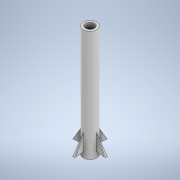
# Autodesk Inventor part: body
Saved by Autodesk Inventor 2022 (Build 260153000, 153)
## iProperties
Created: 2023-01-18
Part Number: body
Material: Generic
Document SubType Name: Modeling
Designer: CLCK
Density: 1 g/cm^3
Appearance: Default
Author: CLCK
Autodesk Inventor part; units mm, degrees
ref_plane "YZ Plane" through (0, 0, 0) normal (1, 0, 0) x (0, 1, 0)
ref_plane "XZ Plane" through (0, 0, 0) normal (0, 1, 0) x (-1, 0, 0)
ref_plane "XY Plane" through (0, 0, 0) normal (0, 0, 1) x (1, 0, 0)
sketch "Sketch2" plane through (0, 0, 0) normal (1, 0, 0) x (0, 1, 0)
  line L0 (50, 4) -> (-50, 4)
  line L1 (-50, 4) -> (-50, -4)
  line L2 (-50, -4) -> (50, -4)
  line L3 (50, -4) -> (50, 4)
  line L4 (50, 4) -> (-50, -4) construction
  line L5 (-50, 4) -> (50, -4) construction
  line L6 (50, 6) -> (-50, 6)
  line L7 (-50, 6) -> (-50, -6)
  line L8 (-50, -6) -> (50, -6)
  line L9 (50, -6) -> (50, 6)
  line L10 (50, 6) -> (-50, -6) construction
  line L11 (-50, 6) -> (50, -6) construction
  line L12 (50, 0) -> (-50, 0)
  point P0 (0, 0)
  dimension "d0" = 100
  dimension "d1" = 8
  dimension "d2" = 100
  dimension "d3" = 12
  constraints: 26 end point, 6 midpoint, 4 parallel, 2 horizontal, 2 perpendicular
  measures "d0" distance of L2.end L1.end
  measures "d1" distance of L1.end L0.end
  measures "d2" distance of L8.end L7.end
  measures "d3" distance of L7.end L6.end
revolve "Revolution1" add sketch "Sketch2" angle 360 about axis through (0, 50, 0) along (0, -1, 0) contours L9 L8 L7 L2
sketch "Sketch4" plane through (0, 0, 0) normal (0, 0, 1) x (1, 0, 0)
  line L0 (6, 50) -> (6, -50) projected
  line L1 (6, -45) -> (6, -30)
  line L2 (6, -30) -> (14.6603, -45)
  line L3 (14.6603, -45) -> (6, -45)
  line L4 (0, 0) -> (0, -56.8241)
  line L5 (4, -50) -> (4, 50) projected
  dimension "d10" = 15
  dimension "d11" = 30
  constraints: 8 end point, 2 point on line, 1 parallel, 1 perpendicular
  measures "d10" distance of L1.start L1.end
  measures "d11" angle of L1 L2
revolve "Revolution3" add sketch "Sketch4" angle 10 mid plane about axis through (0, 0, 0) along (0, -1, 0)
pattern_circular "Circular Pattern1" count 4 over 360 about axis through (0, 0, 0) along (0, -1, 0) of "Revolution3"
fillet "Fillet1" radius 0.5 4 edges at (10.2908, -37.5, -0.9003) (10.2908, -37.5, 0.9003) (10.2908, -45, -0.9003) (10.2908, -45, 0.9003)
fillet "Fillet2" radius 0.5 12 edges at (0.9003, -37.5, -10.2908) (-0.9003, -37.5, -10.2908) (0.9003, -45, -10.2908) (-0.9003, -45, -10.2908) (-10.2908, -37.5, -0.9003) (-10.2908, -37.5, 0.9003) (-10.2908, -45, -0.9003) (-10.2908, -45, 0.9003) (-0.9003, -45, 10.2908) (0.9003, -45, 10.2908) (-0.9003, -37.5, 10.2908) (0.9003, -37.5, 10.2908)
body "Solid1"
